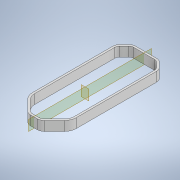
# Autodesk Inventor part: Enclosure Bottom
Saved by Autodesk Inventor 2020 (Build 240168000, 168)
## iProperties
Created: 2021-05-05
Part Number: Enclosure Bottom
Material: Generic
Document SubType Name: Modeling
Designer: Luke
Density: 1 g/cm^3
Appearance: Default
Author: Luke
Autodesk Inventor part; units mm, degrees
ref_plane "YZ Plane" through (0, 0, 0) normal (1, 0, 0) x (0, 1, 0)
ref_plane "XZ Plane" through (0, 0, 0) normal (0, 1, 0) x (-1, 0, 0)
ref_plane "XY Plane" through (0, 0, 0) normal (0, 0, 1) x (1, 0, 0)
sketch "Sketch1" plane through (0, 0, 0) normal (0, 1, 0) x (-1, 0, 0)
  line L0 (-21, -52.5168) -> (-21, 32.4844)
  line L1 (-18.0711, 39.5555) -> (-7.116, 50.5106)
  line L2 (-3.5804, 51.975) -> (3.6277, 51.975)
  line L3 (7.1632, 50.5106) -> (18.0082, 39.6656)
  line L4 (20.9372, 32.5945) -> (20.9371, -52.593)
  line L5 (19.4727, -56.1285) -> (14.6832, -60.918)
  line L6 (11.1477, -62.3824) -> (-11.1267, -62.3824)
  line L7 (-14.6594, -60.9208) -> (-19.5327, -56.0552)
  arc A0 (20.9372, 32.5945) -> (18.0082, 39.6656) centre (10.9372, 32.5945) ccw
  arc A1 (-18.0711, 39.5555) -> (-21, 32.4844) centre (-11, 32.4844) ccw
  arc A2 (-3.5804, 51.975) -> (-7.116, 50.5106) centre (-3.5804, 46.975) ccw
  arc A3 (7.1632, 50.5106) -> (3.6277, 51.975) centre (3.6277, 46.975) ccw
  arc A4 (19.4727, -56.1285) -> (20.9371, -52.593) centre (15.9371, -52.593) ccw
  arc A5 (11.1477, -62.3824) -> (14.6832, -60.918) centre (11.1477, -57.3824) ccw
  arc A6 (-14.6594, -60.9208) -> (-11.1267, -62.3824) centre (-11.1267, -57.3824) ccw
  arc A7 (-21, -52.5168) -> (-19.5327, -56.0552) centre (-16, -52.5168) ccw
  line L8 (-23.0953, 32.4844) -> (-23.0953, -52.5168)
  arc A8 (-23.0953, -52.5168) -> (-21.0132, -57.538) centre (-16, -52.5168) ccw
  line L9 (-21.0132, -57.538) -> (-16.1398, -62.4036)
  arc A9 (-16.1398, -62.4036) -> (-11.1267, -64.4778) centre (-11.1267, -57.3824) ccw
  line L10 (-11.1267, -64.4778) -> (11.1477, -64.4778)
  arc A10 (11.1477, -64.4778) -> (16.1648, -62.3996) centre (11.1477, -57.3824) ccw
  line L11 (16.1648, -62.3996) -> (20.9543, -57.6101)
  arc A11 (20.9543, -57.6101) -> (23.0325, -52.593) centre (15.9371, -52.593) ccw
  line L12 (23.0325, -52.593) -> (23.0325, 32.5945)
  arc A12 (23.0325, 32.5945) -> (19.4898, 41.1472) centre (10.9372, 32.5945) ccw
  line L13 (19.4898, 41.1472) -> (8.6448, 51.9922)
  arc A13 (8.6448, 51.9922) -> (3.6277, 54.0704) centre (3.6277, 46.975) ccw
  line L14 (3.6277, 54.0704) -> (-3.5804, 54.0704)
  arc A14 (-3.5804, 54.0704) -> (-8.5976, 51.9922) centre (-3.5804, 46.975) ccw
  line L15 (-8.5976, 51.9922) -> (-19.5527, 41.0371)
  arc A15 (-19.5527, 41.0371) -> (-23.0953, 32.4844) centre (-11, 32.4844) ccw
  line L16 (-11.9914, -64.4778) -> (12.0086, -64.4778) projected
  point P0 (0, 0)
  point P1 (0, 0)
  point P2 (20.9543, -57.6101)
  dimension "d15" = 2.0953
  constraints: 32 end point, 32 point on circle, 16 centre point
  measures "d15" radial gap between concentric circles of A1 A15
extrude "Extrusion1" add sketch "Sketch1" along normal blind 10
ref_plane "Work Plane5" through (-3.6277, 0, 0.0004) normal (0, 0, 1) x (1, 0, 0)
ref_plane "Work Plane6" through (0.0314, 0, -52.593) normal (-1, 0, 0) x (0, 0, 1)
body "Solid1"
